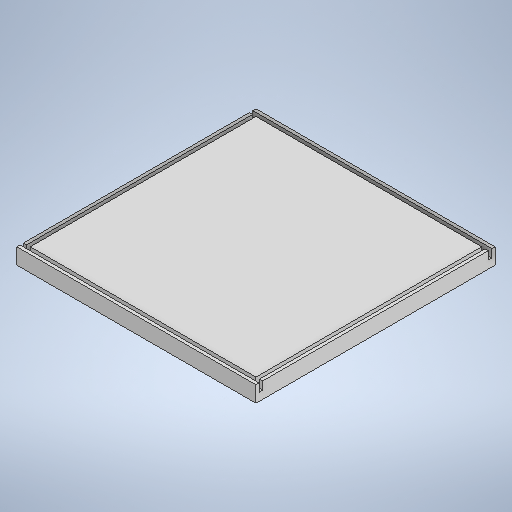
# Autodesk Inventor part: base
Saved by Autodesk Inventor 2026.1 (Build 301233000, 233)
## iProperties
Created: 2026-08-11
Part Number: base
Material: Generic
Document SubType Name: Modeling
Designer: rowan
Density: 1 g/cm^3
Appearance: Default
Author: rowan
Autodesk Inventor part; units mm, degrees
ref_plane "YZ Plane" through (0, 0, 0) normal (1, 0, 0) x (0, 1, 0)
ref_plane "XZ Plane" through (0, 0, 0) normal (0, 1, 0) x (-1, 0, 0)
ref_plane "XY Plane" through (0, 0, 0) normal (0, 0, 1) x (1, 0, 0)
sketch "Sketch1" plane through (0, 0, 0) normal (0, 1, 0) x (-1, 0, 0)
  line L0 (0, 0) -> (150, 0)
  line L1 (150, 0) -> (150, -150)
  line L2 (150, -150) -> (0, -150)
  line L3 (0, -150) -> (0, 0)
  dimension "d0" = 150
  constraints: 8 end point, 2 parallel, 2 perpendicular, 1 horizontal
  measures "d0" distance of L1.end L2.end
extrude "Extrusion1" add sketch "Sketch1" along normal blind 10
sketch "Sketch2" plane through (0, 10, 0) normal (0, 1, 0) x (1, 0, 0)
  line L0 (-150, 2) -> (0, 2)
  line L1 (0, 2) -> (0, 4.2)
  line L2 (0, 4.2) -> (-150, 4.2)
  line L3 (-150, 4.2) -> (-150, 2)
  line L4 (-150, 0) -> (0, 0) projected
  line L5 (-150, 150) -> (-150, 0) projected
  line L6 (-150, 75) -> (0, 75) construction
  line L7 (0, 0) -> (0, 150) projected
  line L8 (-150, 148) -> (0, 148)
  line L9 (0, 148) -> (0, 145.8)
  line L10 (0, 145.8) -> (-150, 145.8)
  line L11 (-150, 145.8) -> (-150, 148)
  line L12 (-148, 4.2) -> (-148, 145.8)
  line L13 (-145.8, 4.2) -> (-145.8, 145.8)
  line L14 (-75, 0) -> (-75, 148) construction
  line L15 (-2, 4.2) -> (-2, 145.8)
  line L16 (-4.2, 4.2) -> (-4.2, 145.8)
  point P0 (0, 148)
  dimension "d3" = 2.2
  dimension "d4" = 2
  dimension "d5" = 2.2
  dimension "d6" = 2
  constraints: 28 end point, 8 symmetric about line, 4 midpoint, 3 parallel, 3 point on line, 2 perpendicular, 1 collinear, 1 horizontal
  measures "d3" distance of L0.end L1.end
  measures "d4" distance between parallel lines of L4 L0
  measures "d5" distance between parallel lines of L12 L13
  measures "d6" distance between parallel lines of L5 L12
extrude "Extrusion2" cut sketch "Sketch2" against normal blind 5 contours L3 L2 L1 L0 | L12 L10 L13 L2 | L5 L8 L7 L10 | L2 L16 L10 L15
body "Solid1"
